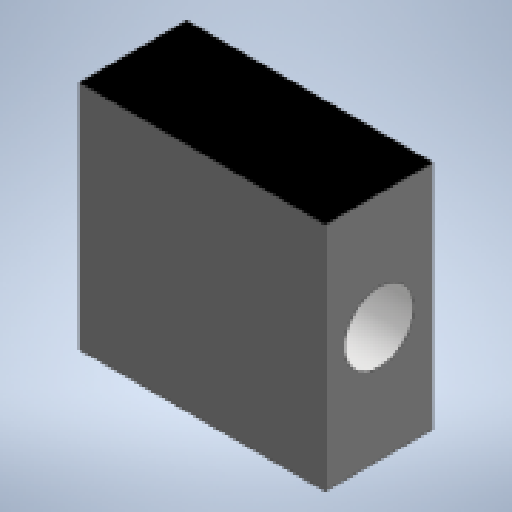
# Autodesk Inventor part: motor on trail
Saved by Autodesk Inventor 2023 (Build 270158000, 158)
## iProperties
Created: 2019-09-11
Part Number: motor on trail
Material: Generic
Document SubType Name: Modeling
Designer: shenglab2
Density: 1 g/cm^3
Appearance: Default
Author: shenglab2
Autodesk Inventor part; units mm, degrees
ref_plane "YZ Plane" through (0, 0, 0) normal (1, 0, 0) x (0, 1, 0)
ref_plane "XZ Plane" through (0, 0, 0) normal (0, 1, 0) x (-1, 0, 0)
ref_plane "XY Plane" through (0, 0, 0) normal (0, 0, 1) x (1, 0, 0)
sketch "Sketch1" plane through (0, 0, 0) normal (0, 0, 1) x (1, 0, 0)
  line L0 (-10.2979, 26.0182) -> (21.7021, 26.0182)
  line L1 (21.7021, 26.0182) -> (21.7021, -3.9818)
  line L2 (21.7021, -3.9818) -> (-10.2979, -3.9818)
  line L3 (-10.2979, -3.9818) -> (-10.2979, 26.0182)
  point P0 (0, 0)
  dimension "d0" = 32
  dimension "d1" = 30
  constraints: 8 end point, 2 parallel, 1 horizontal, 1 perpendicular
  measures "d0" distance of L0.start L0.end
  measures "d1" distance of L0.end L1.end
extrude "Extrusion1" add sketch "Sketch1" along normal blind 14
sketch "Sketch2" plane through (21.7021, -3.9818, 0) normal (1, 0, 0) x (0, 0, -1)
  line L0 (-14, 30) -> (0, 0)
  circle A0 centre (-7, 15) radius 4.5
  point P0 (0, 3.9818)
  dimension "d4" = 9
  constraints: 2 end point, 1 centre point, 1 midpoint
  measures "d4" diameter of A0
extrude "Extrusion2" cut sketch "Sketch2" against normal through all
body "Solid1"
